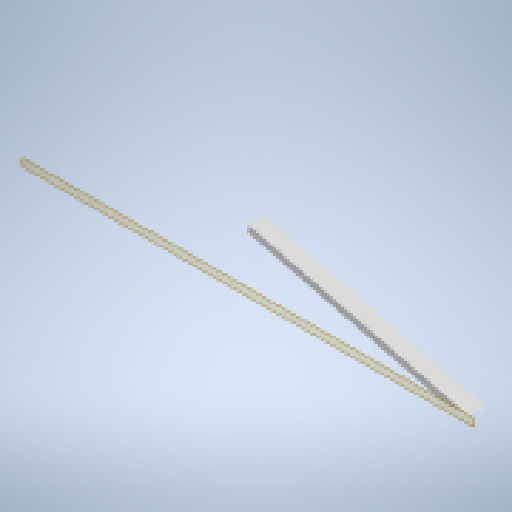
# Autodesk Inventor part: top head slant
Saved by Autodesk Inventor 2025 (Build 290162000, 162)
## iProperties
Created: 2024-09-19
Part Number: top head slant
Material: Generic
Document SubType Name: Modeling
Designer: localadmin
Density: 1 g/cm^3
Appearance: Default
Author: localadmin
Autodesk Inventor part; units mm, degrees
ref_plane "YZ Plane" through (0, 0, 0) normal (1, 0, 0) x (0, 1, 0)
ref_plane "XZ Plane" through (0, 0, 0) normal (0, 1, 0) x (-1, 0, 0)
ref_plane "XY Plane" through (0, 0, 0) normal (0, 0, 1) x (1, 0, 0)
ref_plane "Work Plane1" through (0, 0, 0) normal (0, 0, 1) x (1, 0, 0)
sketch "Sketch1" plane through (0, 0, 0) normal (0, 0, 1) x (1, 0, 0)
  line L0 (-88.9, 0) -> (0, 0) projected
  line L1 (0, 0) -> (0, 38.1) projected
  line L2 (-88.9, 38.1) -> (0, 38.1) projected
  line L3 (-88.9, 0) -> (-88.9, 38.1) projected
  line L4 (0, 0) -> (2260.6, 0) projected
  line L5 (2260.6, 0) -> (2260.6, 38.1) projected
  line L6 (0, 38.1) -> (2260.6, 38.1) projected
  line L7 (0, 0) -> (0, 38.1) projected
  line L8 (2260.6, 0) -> (2349.5, 0) projected
  line L9 (2349.5, 0) -> (2349.5, 38.1) projected
  line L10 (2260.6, 38.1) -> (2349.5, 38.1) projected
  line L11 (2260.6, 0) -> (2260.6, 38.1) projected
  line L12 (1130.3, 38.1) -> (1130.3, 342.9)
  line L13 (1130.3, 342.9) -> (2349.5, 38.1)
  line L14 (1130.3, 342.9) -> (1121.0594, 305.9376)
  line L15 (1121.0594, 305.9376) -> (2192.4097, 38.1)
  point P0 (1130.3, 303.6274)
  dimension "d0" = 304.8
  dimension "d2" = 90
  dimension "d4" = 38.1
  constraints: 8 end point, 1 midpoint, 1 parallel, 1 point on line, 1 vertical
  measures "d0" distance of L12.start L12.end
  measures "d2" angle of L14 L13
  measures "d4" distance between parallel lines of L13 L15
extrude "Extrusion1" add sketch "Sketch1" against normal blind 88.9 contours L6 L15 L12 L13 L10
body "Solid1"
